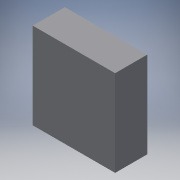
# Autodesk Inventor part: Dummybauteil
Saved by Autodesk Inventor 2018 (Build 220112000, 112)
## iProperties
Created: 2018-01-13
Part Number: Dummybauteil
Material: Generisch
Document SubType Name: Modeling
Designer: gchri
Density: 1 g/cm^3
Appearance: Vorgabe
Author: gchri
Autodesk Inventor part; units mm, degrees
ref_plane "YZ Plane" through (0, 0, 0) normal (1, 0, 0) x (0, 1, 0)
ref_plane "XZ Plane" through (0, 0, 0) normal (0, 1, 0) x (-1, 0, 0)
ref_plane "XY Plane" through (0, 0, 0) normal (0, 0, 1) x (1, 0, 0)
sketch "Skizze1" plane through (0, 0, 0) normal (0, 1, 0) x (-1, 0, 0)
  line L0 (11.3537, 13.7396) -> (-14.3155, 13.7396)
  line L1 (-14.3155, 13.7396) -> (-14.3155, -13.1637)
  line L2 (-14.3155, -13.1637) -> (11.3537, -13.1637)
  line L3 (11.3537, -13.1637) -> (11.3537, 13.7396)
  point P0 (0, 0)
  constraints: 8 end point, 2 parallel, 1 horizontal, 1 perpendicular
extrude "Extrusion1" add sketch "Skizze1" along normal blind 10
